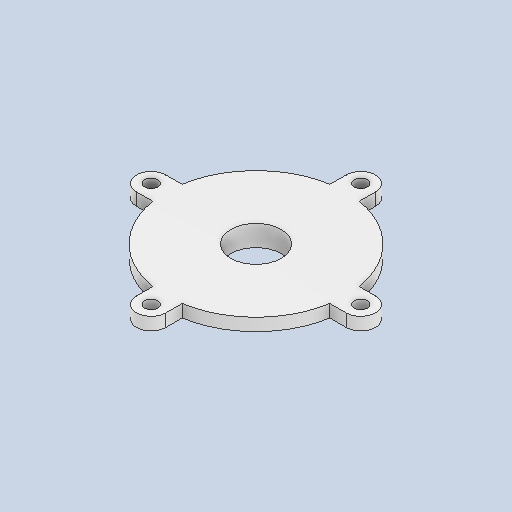
# Autodesk Inventor part: capac_v2
Saved by Autodesk Inventor 2025.2 (Build 292293000, 293)
## iProperties
Created: 2024-01-10
Part Number: capac_v2
Material: Polystyrene
Document SubType Name: Modeling
Designer: mirun
Density: 1.021 g/cm^3
Appearance: Smooth - White
Author: mirun
Autodesk Inventor part; units mm, degrees
ref_plane "YZ Plane" through (0, 0, 0) normal (1, 0, 0) x (0, 1, 0)
ref_plane "XZ Plane" through (0, 0, 0) normal (0, 1, 0) x (-1, 0, 0)
ref_plane "XY Plane" through (0, 0, 0) normal (0, 0, 1) x (1, 0, 0)
sketch "Sketch1" plane through (0, 0, 0) normal (0, 1, 0) x (-1, 0, 0)
  circle A0 centre (0, 0) radius 17.25 construction
  circle A1 centre (0, 0) radius 18.15
  circle A2 centre (0, 0) radius 16.55
  line L0 (0, 0) -> (0, 16.55)
  line L1 (0, 18.15) -> (0, 21.4)
  line L2 (0, 17.25) -> (0, 17.95)
  line L3 (0, 16.55) -> (0, 17.25)
  circle A3 centre (0, 0) radius 17.95 construction
  line L4 (0, 17.95) -> (0, 18.15)
  line L5 (-1, 18.1224) -> (-0.989, 17.9227)
  arc A4 (-0.989, 17.9227) -> (-0.45, 16.5439) centre (1.5045, 18.1027) ccw
  arc A5 (0.45, 16.5439) -> (0.989, 17.9227) centre (-1.5045, 18.1027) ccw
  line L6 (1, 18.1224) -> (0.989, 17.9227)
  circle A6 centre (0, 0) radius 21.4
  line L7 (0, 21.4) -> (0, 22.9158)
  point P0 (0.5157, 15.5846)
  point P1 (0.8657, 17.1732)
  point P2 (0.45, 16.5439)
  point P3 (1, 18.1224)
  dimension "d0" = 34.5
  dimension "d32" = 42.8
  dimension "d1" = 0.7
  dimension "d2" = 0.7
  dimension "d3" = 0.2
  dimension "d4" = 1
  dimension "d5" = 2.5
  dimension "d6" = 0.45
  constraints: 16 end point, 10 point on circle, 6 coincident, 6 vertical, 5 centre point, 4 symmetric about line, 2 vertical alignment, 1 line through centre, 5 other
  measures "d1" distance of L0.end L2.start
  measures "d2" distance of L2.start L2.end
  measures "d3" distance of L1.start L2.end
  measures "d4" horizontal distance of L1.start L5.start
  measures "d5" radius of A4
  measures "d6" horizontal distance of L0.end A2.end
extrude "Extrusion1" add sketch "Sketch1" along normal blind 3 contours A1 L5 A4 A2 A5 L6 | L6 A5 A2 L3 L2 L4 A1 | A1 L4 L2 L3 A2 A4 L5 | A2 | A6
extrude "Extrusion2" add sketch "Sketch1" against normal blind 2 contours A1 L5 A4 A2 A5 L6 | L6 A5 A2 L3 L2 L4 A1 | A1 L4 L2 L3 A2 A4 L5 | A2
extrude "Extrusion3" cut sketch "Sketch1" against normal blind 20 contours L6 A5 A2 L3 L2 L4 A1 | A1 L4 L2 L3 A2 A4 L5
pattern_circular "Circular Pattern2" count 6 over 360 about axis through (0, 0, 0) along (0, 1, 0) of "Extrusion2"
pattern_circular "Circular Pattern3" count 28 over 360 about axis through (0, 0, 0) along (0, -1, 0) of "Extrusion3"
sketch "Sketch2" plane through (0, 0, 0) normal (0, -1, 0) x (1, 0, 0)
  circle A0 centre (0, 0) radius 21.4 construction
  arc A1 (-0.8, 18.3826) -> (-3.3106, 18.0997) centre (0, 0) ccw construction
  circle A2 centre (0, 0) radius 21.4
  circle A3 centre (0, 0) radius 5.95 construction
  circle A4 centre (-25, 0) radius 1.5625
  circle A5 centre (-25, 0) radius 3.5
  line L0 (-25, -3.5) -> (-21.1118, -3.5)
  line L1 (0, 0) -> (0, -27.3802)
  line L2 (0, 0) -> (-32.8745, 0)
  line L3 (-25, 3.5) -> (-21.1118, 3.5)
  point P0 (-18.2315, 1.1897)
  point P1 (-18.2315, 8.1881)
  point P2 (-22.0156, 8.1881)
  point P3 (-11.064, 7.636)
  point P4 (-14.9521, 7.636)
  dimension "d24" = 7
  dimension "d26" = 42.8
  dimension "d23" = 3.125
  dimension "d25" = 25
  constraints: 8 end point, 6 coincident, 3 centre point, 3 horizontal, 2 point on circle, 2 symmetric about line, 1 perpendicular, 1 point on line, 1 vertical, 8 other
  measures "d23" diameter of A4
  measures "d25" distance of point (0, 0) A4.centre
extrude "Extrusion4" add sketch "Sketch2" against normal blind 3 contours A2 L2 A5 L3 | A2 L0 A5 L2 | A5 L2 A4 | A5 L2 A4
pattern_circular "Circular Pattern4" count 4 over 360 about axis through (0, 0, 0) along (0, 1, 0) of "Extrusion4"
extrude "Extrusion5" cut sketch "Sketch1" against normal blind 3 contours L6 A5 A2 L3 L2 L4 A1 | A1 L4 L2 L3 A2 A4 L5
sketch "Sketch3" plane through (0, 3, 0) normal (0, 1, 0) x (1, 0, 0)
  arc A0 (-3.5, 21.1118) -> (-21.1118, 3.5) centre (0, 0) ccw construction
  circle A1 centre (0, 0) radius 6
  dimension "d35" = 12
  constraints: 1 centre point, 1 coincident
  measures "d35" diameter of A1
extrude "Extrusion6" cut sketch "Sketch3" against normal through all
body "Solid1"
